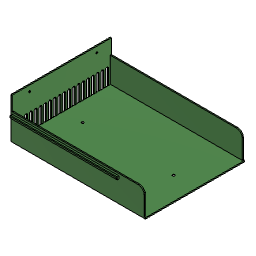
drawer1 (Autodesk Fusion 360 design; units mm, degrees)
Autodesk Fusion 360 part; units mm, degrees
sketch "Skizze1" plane through (0, 0, 0) normal (0, 0, 1) x (1, 0, 0)
  line L0 (5, 5) -> (235, 5)
  line L1 (235, 5) -> (235, 175)
  line L2 (235, 175) -> (5, 175)
  line L3 (5, 175) -> (5, 5)
  dimension "d1" = 230
  dimension "d2" = 170
  constraint horizontal L0
  constraint vertical L1
  constraint horizontal L2
  constraint vertical L3
  measures "d1" distance of L0.start L0.end
  measures "d2" distance of L0.start L2.end
extrude "Extrusion1" add sketch "Skizze1" along normal blind 45
shell "Schale1" thickness 2 removed faces 1 at (81.6667, 61.6667, 45)
sketch "Skizze2" plane through (0, 0, 45) normal (0, 0, 1) x (-1, 0, 0)
  line L0 (-7, -173) -> (-233, -173)
  line L1 (-233, -173) -> (-233, -7)
  line L2 (-233, -7) -> (-7, -7)
  line L3 (-7, -7) -> (-7, -173)
  line L4 (-5, -175) -> (-5, -5)
  line L5 (-5, -5) -> (-235, -5)
  line L6 (-235, -5) -> (-235, -175)
  line L7 (-235, -175) -> (-5, -175)
  line L8 (-7, -173) -> (-7, -175)
  line L9 (-7, -7) -> (-7, -5)
  constraint coincident L0.start L3.end
  constraint perpendicular L0 L8
  constraint coincident L2.end L3.start
  constraint coincident L5 L9.end
  constraint perpendicular L5 L9
extrude "Extrusion2" add sketch "Skizze2" along normal blind 25 contours L3 L4 L5 L7 L8 L9
sketch "Skizze3" plane through (0, 0, 45) normal (0, 0, 1) x (-1, 0, 0)
  line L0 (-7, -175) -> (-7, -173)
  line L1 (-7, -173) -> (-233, -173)
  line L2 (-233, -173) -> (-233, -7)
  line L3 (-233, -7) -> (-7, -7)
  line L4 (-7, -7) -> (-7, -5)
  line L5 (-7, -5) -> (-235, -5)
  line L6 (-235, -5) -> (-235, -175)
  line L7 (-235, -175) -> (-7, -175)
  line L8 (-233, -7) -> (-233, -5)
  line L9 (-233, -173) -> (-233, -175)
  constraint coincident L2.end L3.start
  constraint coincident L5 L8.end
  constraint perpendicular L5 L8
  constraint coincident L1.end L2.start
  constraint coincident L7 L9.end
  constraint perpendicular L7 L9
extrude "Extrusion3" cut sketch "Skizze3" against normal blind 20 contours L2 L5 L6 L7 L8 L9
fillet "Abrundung1" radius 10 1 edges at (233, 6, 45)
fillet "Abrundung2" radius 10 1 edges at (233, 174, 45)
sketch "Skizze4" plane through (0, 5, 0) normal (0, -1, 0) x (1, 0, 0)
  arc A0 (233, 35) -> (223, 45) centre (223, 35) ccw
  line L0 (223, 45) -> (7, 45)
  line L1 (7, 45) -> (7, 70)
  line L2 (7, 70) -> (5, 70)
  line L3 (5, 70) -> (5, 0)
  line L4 (5, 0) -> (235, 0)
  line L5 (235, 0) -> (235, 25)
  line L6 (235, 25) -> (233, 25)
  line L7 (233, 25) -> (233, 35)
  line L8 (7, 0) -> (7, 37) construction
  line L9 (190, 0) -> (190, 37) construction
  line L10 (7, 37) -> (190, 37)
  line L11 (7, 41.5) -> (190, 41.5)
  line L12 (7, 41.5) -> (7, 37)
  line L13 (190, 41.5) -> (190, 37)
  dimension "d16" = 37
  dimension "d17" = 37
  dimension "d25" = 183
  constraint coincident L4 L8.start
  constraint perpendicular L4 L8
  constraint perpendicular L9 L10
  constraint perpendicular L10 L12
  constraint perpendicular L10 L13
  measures "d16" distance of L8.start L8.end
  measures "d17" distance of L9.end L9.start
  measures "d25" distance of L11.start L11.end
extrude "Extrusion4" add sketch "Skizze4" along normal blind 4 contours L10 L11 L12 L13
chamfer "Fase1" distance 1 angle 45 2 edges at (98.5, 1, 41.5) (98.5, 1, 37)
fillet "Abrundung3" radius 1 1 edges at (190, 1, 39.25)
sketch "Skizze5" plane through (0, 175, 0) normal (0, 1, 0) x (-1, 0, 0)
  arc A0 (-223, 45) -> (-233, 35) centre (-223, 35) ccw
  line L0 (-233, 35) -> (-233, 25)
  line L1 (-233, 25) -> (-235, 25)
  line L2 (-235, 25) -> (-235, 0)
  line L3 (-235, 0) -> (-5, 0)
  line L4 (-5, 0) -> (-5, 70)
  line L5 (-5, 70) -> (-7, 70)
  line L6 (-7, 70) -> (-7, 45)
  line L7 (-7, 45) -> (-223, 45)
  line L8 (-6.7409, 0) -> (-6.7409, 37) construction
  line L9 (-189.7409, 0) -> (-189.7409, 37) construction
  line L10 (-189.7409, 37) -> (-6.7409, 37)
  line L11 (-189.7409, 41.5) -> (-6.7409, 41.5)
  line L12 (-189.7409, 41.5) -> (-189.7409, 37)
  line L13 (-6.7409, 41.5) -> (-6.7409, 37)
  dimension "d23" = 37
  dimension "d26" = 37
  constraint coincident L3 L8.start
  constraint perpendicular L3 L8
  constraint perpendicular L8 L10
  constraint perpendicular L10 L12
  constraint perpendicular L10 L13
  measures "d23" distance of L8.start L8.end
  measures "d26" distance of L9.end L9.start
extrude "Extrusion5" add sketch "Skizze5" along normal blind 4.5 contours L10 L11 L12 L13
chamfer "Fase2" distance 1 angle 45 2 edges at (98.2409, 179.5, 41.5) (98.2409, 179.5, 37)
fillet "Abrundung4" radius 1 1 edges at (189.7409, 179.5, 39.25)
sketch "Skizze6" plane through (5, 0, 0) normal (-1, 0, 0) x (0, -1, 0)
  line L0 (-175, 0) -> (-5, 0)
  line L1 (-5, 0) -> (-5, 70)
  line L2 (-5, 70) -> (-175, 70)
  line L3 (-175, 70) -> (-175, 0)
sketch "Skizze7" plane through (5, 0, 0) normal (-1, 0, 0) x (0, -1, 0)
  line L0 (-175, 70) -> (-175, 60) construction
  line L1 (-5, 70) -> (-5, 60) construction
  line L2 (-175, 60) -> (-5, 60) construction
  circle A0 centre (-150, 60) radius 1.5
  circle A1 centre (-35, 60) radius 1.5
  point P0 (-35, 60)
  dimension "d32" = 10
  dimension "d33" = 10
  dimension "d34" = 3
  dimension "d37" = 115
  dimension "d38" = 0
  dimension "d39" = 3
  constraint vertical L0
  constraint vertical L1
  constraint perpendicular L1 L2
  constraint coincident L2 A0.centre
  constraint coincident P0 A1.centre
  measures "d32" distance of L0.start L0.end
  measures "d33" distance of L1.start L1.end
  measures "d34" diameter of A0
  measures "d39" diameter of A1
hole "Bohrung1" at (5, 150, 60) at (5, 35, 60) direction (1, 0, 0) diameter 3 depth 2 tip angle 180 countersink diameter 6 countersink angle 90
sketch "Skizze8" plane through (0, 0, 0) normal (0, 0, -1) x (1, 0, 0)
  line L0 (5, -5) -> (5, -175)
  line L1 (5, -175) -> (235, -175)
  line L2 (235, -175) -> (235, -5)
  line L3 (235, -5) -> (5, -5)
  line L4 (8.1647, -9.2838) -> (228.1647, -9.2838) construction
  line L5 (228.1647, -9.2838) -> (228.1647, -124.2838) construction
  line L6 (228.1647, -124.2838) -> (8.1647, -124.2838) construction
  line L7 (8.1647, -124.2838) -> (8.1647, -9.2838) construction
  line L8 (40.1647, -124.2838) -> (40.1647, -9.2838) construction
  line L9 (196.1647, -9.2838) -> (196.1647, -124.2838) construction
  line L10 (228.1647, -92.2838) -> (8.1647, -92.2838) construction
  line L11 (8.1647, -41.2838) -> (228.1647, -41.2838) construction
  circle A0 centre (40.1647, -92.2838) radius 2
  circle A1 centre (196.1647, -92.2838) radius 2
  circle A2 centre (40.1647, -41.2838) radius 2
  circle A3 centre (196.1647, -41.2838) radius 2
  dimension "d45" = 220
  dimension "d46" = 115
  dimension "d51" = 115
  dimension "d52" = 220
  dimension "d53" = 4
  dimension "d54" = 4
  dimension "d55" = 4
  dimension "d56" = 4
  constraint horizontal L4
  constraint vertical L5
  constraint horizontal L6
  constraint vertical L7
  constraint vertical L8
  constraint vertical L9
  constraint horizontal L10
  constraint horizontal L11
  constraint coincident L8 A0.centre
  constraint coincident L10 A0.centre
  constraint coincident L9 A1.centre
  constraint coincident L10 A1.centre
  constraint coincident L8 A2.centre
  constraint coincident L11 A2.centre
  constraint coincident L9 A3.centre
  constraint coincident L11 A3.centre
  measures "d45" distance of L4.start L4.end
  measures "d46" distance of L4.start L6.end
  measures "d51" distance of L8.end L8.start
  measures "d52" distance of L11.start L11.end
  measures "d53" diameter of A0
  measures "d54" diameter of A1
  measures "d55" diameter of A2
  measures "d56" diameter of A3
extrude "Extrusion7" cut 1 faces at (234.3333, 62.3333, 25) along direction (0, 0, -1) blind 23
hole "Bohrung2" at (40.1647, 92.2838, 0) at (196.1647, 92.2838, 0) at (196.1647, 41.2838, 0) at (40.1647, 41.2838, 0) direction (0, 0, 1) diameter 4 depth 3.3 tip angle 180 countersink diameter 8 countersink angle 90
sketch "Skizze9" plane through (5, 0, 0) normal (-1, 0, 0) x (0, -1, 0)
  circle A0 centre (-150, 60) radius 3
  circle A1 centre (-35, 60) radius 3
  line L0 (-175, 0) -> (-5, 0)
  line L1 (-5, 0) -> (-5, 70)
  line L2 (-5, 70) -> (-175, 70)
  line L3 (-175, 70) -> (-175, 0)
  line L4 (-170, 0) -> (-165, 0)
  line L5 (-165, 0) -> (-165, 28)
  line L6 (-167, 30) -> (-168, 30)
  line L7 (-170, 28) -> (-170, 0)
  arc A2 (-168, 30) -> (-170, 28) centre (-168, 28) ccw
  arc A3 (-165, 28) -> (-167, 30) centre (-167, 28) ccw
  line L8 (-161.8421, 0) -> (-156.8421, 0)
  arc A4 (-156.8421, 28) -> (-158.8421, 30) centre (-158.8421, 28) ccw
  line L9 (-158.8421, 30) -> (-159.8421, 30)
  line L10 (-156.8421, 0) -> (-156.8421, 28)
  line L11 (-161.8421, 28) -> (-161.8421, 0)
  arc A5 (-159.8421, 30) -> (-161.8421, 28) centre (-159.8421, 28) ccw
  line L12 (-166.8421, 0) -> (3.1579, 0)
  line L13 (-153.6842, 0) -> (-148.6842, 0)
  arc A6 (-148.6842, 28) -> (-150.6842, 30) centre (-150.6842, 28) ccw
  line L14 (-150.6842, 30) -> (-151.6842, 30)
  line L15 (-148.6842, 0) -> (-148.6842, 28)
  line L16 (-153.6842, 28) -> (-153.6842, 0)
  arc A7 (-151.6842, 30) -> (-153.6842, 28) centre (-151.6842, 28) ccw
  line L17 (-158.6842, 0) -> (11.3158, 0)
  line L18 (-145.5263, 0) -> (-140.5263, 0)
  arc A8 (-140.5263, 28) -> (-142.5263, 30) centre (-142.5263, 28) ccw
  line L19 (-142.5263, 30) -> (-143.5263, 30)
  line L20 (-140.5263, 0) -> (-140.5263, 28)
  line L21 (-145.5263, 28) -> (-145.5263, 0)
  arc A9 (-143.5263, 30) -> (-145.5263, 28) centre (-143.5263, 28) ccw
  line L22 (-150.5263, 0) -> (19.4737, 0)
  line L23 (-137.3684, 0) -> (-132.3684, 0)
  arc A10 (-132.3684, 28) -> (-134.3684, 30) centre (-134.3684, 28) ccw
  line L24 (-134.3684, 30) -> (-135.3684, 30)
  line L25 (-132.3684, 0) -> (-132.3684, 28)
  line L26 (-137.3684, 28) -> (-137.3684, 0)
  arc A11 (-135.3684, 30) -> (-137.3684, 28) centre (-135.3684, 28) ccw
  line L27 (-142.3684, 0) -> (27.6316, 0)
  line L28 (-129.2105, 0) -> (-124.2105, 0)
  arc A12 (-124.2105, 28) -> (-126.2105, 30) centre (-126.2105, 28) ccw
  line L29 (-126.2105, 30) -> (-127.2105, 30)
  line L30 (-124.2105, 0) -> (-124.2105, 28)
  line L31 (-129.2105, 28) -> (-129.2105, 0)
  arc A13 (-127.2105, 30) -> (-129.2105, 28) centre (-127.2105, 28) ccw
  line L32 (-134.2105, 0) -> (35.7895, 0)
  line L33 (-121.0526, 0) -> (-116.0526, 0)
  arc A14 (-116.0526, 28) -> (-118.0526, 30) centre (-118.0526, 28) ccw
  line L34 (-118.0526, 30) -> (-119.0526, 30)
  line L35 (-116.0526, 0) -> (-116.0526, 28)
  line L36 (-121.0526, 28) -> (-121.0526, 0)
  arc A15 (-119.0526, 30) -> (-121.0526, 28) centre (-119.0526, 28) ccw
  line L37 (-126.0526, 0) -> (43.9474, 0)
  line L38 (-112.8947, 0) -> (-107.8947, 0)
  arc A16 (-107.8947, 28) -> (-109.8947, 30) centre (-109.8947, 28) ccw
  line L39 (-109.8947, 30) -> (-110.8947, 30)
  line L40 (-107.8947, 0) -> (-107.8947, 28)
  line L41 (-112.8947, 28) -> (-112.8947, 0)
  arc A17 (-110.8947, 30) -> (-112.8947, 28) centre (-110.8947, 28) ccw
  line L42 (-117.8947, 0) -> (52.1053, 0)
  line L43 (-104.7368, 0) -> (-99.7368, 0)
  arc A18 (-99.7368, 28) -> (-101.7368, 30) centre (-101.7368, 28) ccw
  line L44 (-101.7368, 30) -> (-102.7368, 30)
  line L45 (-99.7368, 0) -> (-99.7368, 28)
  line L46 (-104.7368, 28) -> (-104.7368, 0)
  arc A19 (-102.7368, 30) -> (-104.7368, 28) centre (-102.7368, 28) ccw
  line L47 (-109.7368, 0) -> (60.2632, 0)
  line L48 (-96.5789, 0) -> (-91.5789, 0)
  arc A20 (-91.5789, 28) -> (-93.5789, 30) centre (-93.5789, 28) ccw
  line L49 (-93.5789, 30) -> (-94.5789, 30)
  line L50 (-91.5789, 0) -> (-91.5789, 28)
  line L51 (-96.5789, 28) -> (-96.5789, 0)
  arc A21 (-94.5789, 30) -> (-96.5789, 28) centre (-94.5789, 28) ccw
  line L52 (-101.5789, 0) -> (68.4211, 0)
  line L53 (-88.4211, 0) -> (-83.4211, 0)
  arc A22 (-83.4211, 28) -> (-85.4211, 30) centre (-85.4211, 28) ccw
  line L54 (-85.4211, 30) -> (-86.4211, 30)
  line L55 (-83.4211, 0) -> (-83.4211, 28)
  line L56 (-88.4211, 28) -> (-88.4211, 0)
  arc A23 (-86.4211, 30) -> (-88.4211, 28) centre (-86.4211, 28) ccw
  line L57 (-93.4211, 0) -> (76.5789, 0)
  line L58 (-80.2632, 0) -> (-75.2632, 0)
  arc A24 (-75.2632, 28) -> (-77.2632, 30) centre (-77.2632, 28) ccw
  line L59 (-77.2632, 30) -> (-78.2632, 30)
  line L60 (-75.2632, 0) -> (-75.2632, 28)
  line L61 (-80.2632, 28) -> (-80.2632, 0)
  arc A25 (-78.2632, 30) -> (-80.2632, 28) centre (-78.2632, 28) ccw
  line L62 (-85.2632, 0) -> (84.7368, 0)
  line L63 (-72.1053, 0) -> (-67.1053, 0)
  arc A26 (-67.1053, 28) -> (-69.1053, 30) centre (-69.1053, 28) ccw
  line L64 (-69.1053, 30) -> (-70.1053, 30)
  line L65 (-67.1053, 0) -> (-67.1053, 28)
  line L66 (-72.1053, 28) -> (-72.1053, 0)
  arc A27 (-70.1053, 30) -> (-72.1053, 28) centre (-70.1053, 28) ccw
  line L67 (-77.1053, 0) -> (92.8947, 0)
  line L68 (-63.9474, 0) -> (-58.9474, 0)
  arc A28 (-58.9474, 28) -> (-60.9474, 30) centre (-60.9474, 28) ccw
  line L69 (-60.9474, 30) -> (-61.9474, 30)
  line L70 (-58.9474, 0) -> (-58.9474, 28)
  line L71 (-63.9474, 28) -> (-63.9474, 0)
  arc A29 (-61.9474, 30) -> (-63.9474, 28) centre (-61.9474, 28) ccw
  line L72 (-68.9474, 0) -> (101.0526, 0)
  line L73 (-55.7895, 0) -> (-50.7895, 0)
  arc A30 (-50.7895, 28) -> (-52.7895, 30) centre (-52.7895, 28) ccw
  line L74 (-52.7895, 30) -> (-53.7895, 30)
  line L75 (-50.7895, 0) -> (-50.7895, 28)
  line L76 (-55.7895, 28) -> (-55.7895, 0)
  arc A31 (-53.7895, 30) -> (-55.7895, 28) centre (-53.7895, 28) ccw
  line L77 (-60.7895, 0) -> (109.2105, 0)
  line L78 (-47.6316, 0) -> (-42.6316, 0)
  arc A32 (-42.6316, 28) -> (-44.6316, 30) centre (-44.6316, 28) ccw
  line L79 (-44.6316, 30) -> (-45.6316, 30)
  line L80 (-42.6316, 0) -> (-42.6316, 28)
  line L81 (-47.6316, 28) -> (-47.6316, 0)
  arc A33 (-45.6316, 30) -> (-47.6316, 28) centre (-45.6316, 28) ccw
  line L82 (-52.6316, 0) -> (117.3684, 0)
  line L83 (-39.4737, 0) -> (-34.4737, 0)
  arc A34 (-34.4737, 28) -> (-36.4737, 30) centre (-36.4737, 28) ccw
  line L84 (-36.4737, 30) -> (-37.4737, 30)
  line L85 (-34.4737, 0) -> (-34.4737, 28)
  line L86 (-39.4737, 28) -> (-39.4737, 0)
  arc A35 (-37.4737, 30) -> (-39.4737, 28) centre (-37.4737, 28) ccw
  line L87 (-44.4737, 0) -> (125.5263, 0)
  line L88 (-31.3158, 0) -> (-26.3158, 0)
  arc A36 (-26.3158, 28) -> (-28.3158, 30) centre (-28.3158, 28) ccw
  line L89 (-28.3158, 30) -> (-29.3158, 30)
  line L90 (-26.3158, 0) -> (-26.3158, 28)
  line L91 (-31.3158, 28) -> (-31.3158, 0)
  arc A37 (-29.3158, 30) -> (-31.3158, 28) centre (-29.3158, 28) ccw
  line L92 (-36.3158, 0) -> (133.6842, 0)
  line L93 (-23.1579, 0) -> (-18.1579, 0)
  arc A38 (-18.1579, 28) -> (-20.1579, 30) centre (-20.1579, 28) ccw
  line L94 (-20.1579, 30) -> (-21.1579, 30)
  line L95 (-18.1579, 0) -> (-18.1579, 28)
  line L96 (-23.1579, 28) -> (-23.1579, 0)
  arc A39 (-21.1579, 30) -> (-23.1579, 28) centre (-21.1579, 28) ccw
  line L97 (-28.1579, 0) -> (141.8421, 0)
  line L98 (-15, 0) -> (-10, 0)
  arc A40 (-10, 28) -> (-12, 30) centre (-12, 28) ccw
  line L99 (-12, 30) -> (-13, 30)
  line L100 (-10, 0) -> (-10, 28)
  line L101 (-15, 28) -> (-15, 0)
  arc A41 (-13, 30) -> (-15, 28) centre (-13, 28) ccw
  line L102 (-20, 0) -> (150, 0)
  dimension "d62" = 2
  dimension "d63" = 2
  dimension "d66" = 155
  dimension "d67" = 0
  constraint horizontal L4
  constraint vertical L5
  constraint horizontal L6
  constraint vertical L7
  constraint coincident L0 L4.start
  constraint tangent L6 A2
  constraint tangent L7 A2
  constraint tangent L5 A3
  constraint tangent L6 A3
  measures "d62" radius of A2
  measures "d63" radius of A3
extrude "Extrusion8" cut sketch "Skizze9" against normal blind 2 contours L0 L4 L5 L6 L7 A2 A3 L12 | L0 L8 A4 L9 L10 L11 A5 L12 L17 | L0 L12 L17 L22 L27 L32 L37 L42 L47 L52 L57 L62 L67 L72 L77 L82 L87 L92 L97 L98 A40 L99 L100 L101 A41 L102 | L0 L12 L17 L22 L27 L32 L37 L42 L47 L52 L57 L62 L67 L72 L77 L82 L87 L92 L93 A38 L94 L95 L96 A39 L97 L102 | L0 L12 L13 A6 L14 L15 L16 A7 L17 L22 | L0 L12 L17 L22 L27 L32 L37 L42 L47 L52 L57 L62 L67 L72 L77 L82 L87 L88 A36 L89 L90 L91 A37 L92 L97 | L0 L12 L17 L18 A8 L19 L20 L21 A9 L22 L27 | L0 L12 L17 L22 L27 L32 L37 L42 L47 L52 L57 L62 L67 L72 L77 L82 L83 A34 L84 L85 L86 A35 L87 L92 | L0 L12 L17 L22 L23 A10 L24 L25 L26 A11 L27 L32 | L0 L12 L17 L22 L27 L32 L37 L42 L47 L52 L57 L62 L67 L72 L77 L78 A32 L79 L80 L81 A33 L82 L87 | L0 L12 L17 L22 L27 L28 A12 L29 L30 L31 A13 L32 L37 | L0 L12 L17 L22 L27 L32 L37 L42 L47 L52 L57 L62 L67 L72 L73 A30 L74 L75 L76 A31 L77 L82 | L0 L12 L17 L22 L27 L32 L33 A14 L34 L35 L36 A15 L37 L42 | L0 L12 L17 L22 L27 L32 L37 L42 L47 L52 L57 L62 L67 L68 A28 L69 L70 L71 A29 L72 L77 | L0 L12 L17 L22 L27 L32 L37 L38 A16 L39 L40 L41 A17 L42 L47 | L0 L12 L17 L22 L27 L32 L37 L42 L47 L52 L57 L62 L63 A26 L64 L65 L66 A27 L67 L72 | L0 L12 L17 L22 L27 L32 L37 L42 L43 A18 L44 L45 L46 A19 L47 L52 | L0 L12 L17 L22 L27 L32 L37 L42 L47 L52 L57 L58 A24 L59 L60 L61 A25 L62 L67 | L0 L12 L17 L22 L27 L32 L37 L42 L47 L48 A20 L49 L50 L51 A21 L52 L57 | L0 L12 L17 L22 L27 L32 L37 L42 L47 L52 L53 A22 L54 L55 L56 A23 L57 L62
extrude "Extrusion6" [suppressed]
